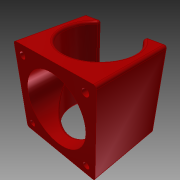
# Autodesk Inventor part: hotend_cooling_mount
Saved by Autodesk Inventor 2014 (Build 180170000, 170)
## iProperties
Created: 2014-03-26
Part Number: hotend_cooling_mount
Material: ABS Plastic
Document SubType Name: Modeling
Designer: buben
Density: 1.06 g/cm^3
Appearance: Smooth - Red
Author: buben
Autodesk Inventor part; units mm, degrees
ref_plane "YZ Plane" through (0, 0, 0) normal (1, 0, 0) x (0, 1, 0)
ref_plane "XZ Plane" through (0, 0, 0) normal (0, 1, 0) x (-1, 0, 0)
sketch "Sketch1" plane through (0, 0, 0) normal (0, 1, 0) x (-1, 0, 0)
  line L0 (0, 0) -> (-32, 0)
  line L1 (-32, 0) -> (-32, -32)
  line L2 (-32, -32) -> (0, -32)
  line L3 (0, -32) -> (0, 0)
  dimension "d0" = 32
  constraints: 8 end point, 2 parallel, 2 perpendicular, 1 horizontal
  measures "d0" distance of L0.start L0.end
extrude "Extrusion1" add sketch "Sketch1" along normal blind 28
sketch "Sketch2" plane through (0, 0, 0) normal (0, 0, 1) x (1, 0, 0)
  line L0 (0, 0) -> (32, 0) projected
  line L1 (0, 28) -> (32, 28) projected
  arc A0 (9.0502, 28) -> (22.9498, 28) centre (16, 17.55) ccw
  point P0 (16, 0)
  dimension "d3" = 25.1
  dimension "d4" = 17.55
  constraints: 2 point on circle, 2 point on line, 1 centre point, 1 midpoint, 1 vertical alignment
  measures "d3" diameter of A0
  measures "d4" distance of point (16, 0) A0.centre
extrude "Extrusion2" cut sketch "Sketch2" against normal through all
ref_plane "Work Plane1" through (16, 17.55, 0) normal (0, -1, 0) x (1, 0, 0)
sketch "Sketch3" plane through (0, 0, 0) normal (0, -1, 0) x (1, 0, 0)
  line L0 (0, 0) -> (32, 0) projected
  line L1 (32, 0) -> (32, -32) projected
  circle A0 centre (16, -16) radius 12.5
  point P0 (16, 0)
  point P1 (32, -16)
  dimension "d7" = 25
  constraints: 2 midpoint, 1 centre point, 1 horizontal alignment, 1 vertical alignment
  measures "d7" diameter of A0
extrude "Extrusion3" cut sketch "Sketch3" against normal up to surface (17.55 mm away)
sketch "Sketch4" plane through (0, 0, 0) normal (0, -1, 0) x (1, 0, 0)
  circle A0 centre (16, -16) radius 12.5 projected
  line L0 (3.5, -3.5) -> (28.5, -3.5) construction
  line L1 (28.5, -3.5) -> (28.5, -28.5) construction
  line L2 (28.5, -28.5) -> (3.5, -28.5) construction
  line L3 (3.5, -28.5) -> (3.5, -3.5) construction
  point P0 (16, -3.5)
  point P1 (28.5, -16)
  dimension "d10" = 25
  constraints: 8 end point, 4 coincident, 2 midpoint, 2 parallel, 2 perpendicular, 1 horizontal, 1 horizontal alignment, 1 vertical alignment
  measures "d10" distance of L1.end L2.end
hole "Hole1" at (3.5, 0, -3.5) at (28.5, 0, -3.5) at (28.5, 0, -28.5) at (3.5, 0, -28.5) direction (0, 1, 0) diameter 2.5 depth 8 tip angle 90
fillet "Fillet1" radius 1 14 edges at (0, 14, 0) (32, 14, 0) (32, 14, -32) (0, 14, -32) (4.5251, 28, 0) (0, 28, -16) (4.5251, 28, -32) (27.4749, 28, -32) (32, 28, -16) (27.4749, 28, 0) (9.0502, 28, -16) (22.9498, 28, -16) (16, 5, 0) (16, 5, -32)
fillet "Fillet2" radius 0.8 1 edges at (3.5277, 16.1555, -16.8319)
body "Solid1"
